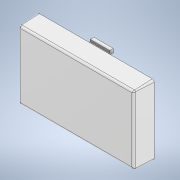
# Autodesk Inventor part: case_up
Saved by Autodesk Inventor 2022 (Build 260153000, 153)
## iProperties
Created: 2022-01-08
Part Number: case_up
Material: Пластик АБС
Document SubType Name: Modeling
Designer: Me
Density: 1.06 g/cm^3
Appearance: Гладкий — белый
Author: Me
Autodesk Inventor part; units mm, degrees
ref_plane "YZ Plane" through (0, 0, 0) normal (1, 0, 0) x (0, 1, 0)
ref_plane "XZ Plane" through (0, 0, 0) normal (0, 1, 0) x (-1, 0, 0)
ref_plane "XY Plane" through (0, 0, 0) normal (0, 0, 1) x (1, 0, 0)
sketch "Эскиз1" plane through (0, 0, 0) normal (0, 0, 1) x (1, 0, 0)
  line L0 (-29, 18) -> (29, 18)
  line L1 (30, 17) -> (30, -17)
  line L2 (29, -18) -> (-29, -18)
  line L3 (-30, -17) -> (-30, 17)
  arc A0 (-29, 18) -> (-30, 17) centre (-29, 17) ccw
  arc A1 (-30, -17) -> (-29, -18) centre (-29, -17) ccw
  arc A2 (29, -18) -> (30, -17) centre (29, -17) ccw
  arc A3 (30, 17) -> (29, 18) centre (29, 17) ccw
  point P0 (0, 0)
  point P1 (-30, 18)
  point P2 (30, 18)
  point P3 (-30, -18)
  dimension "d0" = 60
  dimension "d1" = 36
  dimension "d2" = 18
  dimension "d3" = 30
  dimension "d4" = 1
  constraints: 8 end point, 8 point on circle, 8 tangent, 6 point on line, 4 centre point, 3 equal radius, 2 parallel, 1 horizontal, 1 perpendicular
  measures "d0" distance of point (-30, 18) point (30, 18)
  measures "d1" distance of point (-30, -18) point (-30, 18)
  measures "d2" distance from line of point (0, 0) L0
  measures "d3" distance from line of point (0, 0) L1
  measures "d4" radius of A0
extrude "Выдавливание1" add sketch "Эскиз1" along normal blind 4
sketch "Эскиз3" plane through (0, 0, 4) normal (0, 0, 1) x (1, 0, 0)
  line L0 (-29, 18) -> (29, 18)
  line L1 (30, 17) -> (30, -17)
  line L2 (29, -18) -> (-29, -18)
  line L3 (-30, -17) -> (-30, 17)
  line L4 (30, -17) -> (30, 17) projected
  line L5 (-29, -18) -> (29, -18) projected
  line L6 (-30, 17) -> (-30, -17) projected
  line L7 (29, 18) -> (-29, 18) projected
  arc A0 (-29, 18) -> (-30, 17) centre (-29, 17) ccw
  arc A1 (-30, -17) -> (-29, -18) centre (-29, -17) ccw
  arc A2 (29, -18) -> (30, -17) centre (29, -17) ccw
  arc A3 (30, 17) -> (29, 18) centre (29, 17) ccw
  point P0 (0, 0)
  dimension "d7" = 0
  dimension "d8" = 0
  dimension "d9" = 0
  dimension "d10" = 0
  dimension "d11" = 1
  constraints: 8 end point, 8 point on circle, 8 tangent, 4 centre point, 3 equal radius, 2 parallel, 1 horizontal, 1 perpendicular
  measures "d7" distance between parallel lines of L4 L1
  measures "d8" distance between parallel lines of L5 L2
  measures "d9" distance between parallel lines of L6 L3
  measures "d10" distance between parallel lines of L7 L0
  measures "d11" radius of A0
extrude "Выдавливание2" add sketch "Эскиз3" along normal blind 10 draft -3
sketch "Эскиз4" plane through (0, 0, 0) normal (0, 0, -1) x (-1, 0, 0)
  line L0 (-27.5, 15.5) -> (27.5, 15.5)
  line L1 (27.5, 15.5) -> (27.5, -15.5)
  line L2 (27.5, -15.5) -> (-27.5, -15.5)
  line L3 (-27.5, -15.5) -> (-27.5, 15.5)
  point P0 (0, 0)
  dimension "d14" = 15.5
  dimension "d15" = 31
  dimension "d16" = 27.5
  dimension "d17" = 55
  constraints: 8 end point, 2 parallel, 1 horizontal, 1 perpendicular
  measures "d14" distance from line of point (0, 0) L0
  measures "d15" distance of L0.end L1.end
  measures "d16" distance from line of point (0, 0) L1
  measures "d17" distance of L0.start L0.end
extrude "Выдавливание3" cut sketch "Эскиз4" against normal blind 13 draft -3
sketch "Эскиз5" plane through (0, 0, 0) normal (0, 0, -1) x (-1, 0, 0)
  line L0 (-28.5, 16.5) -> (28.5, 16.5)
  line L1 (28.5, 16.5) -> (28.5, -16.5)
  line L2 (28.5, -16.5) -> (-28.5, -16.5)
  line L3 (-28.5, -16.5) -> (-28.5, 16.5)
  line L4 (-29, 18) -> (29, 18) projected
  line L5 (-30, -17) -> (-30, 17) projected
  line L6 (29, -18) -> (-29, -18) projected
  line L7 (30, 17) -> (30, -17) projected
  line L8 (-29, 18) -> (29, 18)
  line L9 (30, 17) -> (30, -17)
  line L10 (29, -18) -> (-29, -18)
  line L11 (-30, -17) -> (-30, 17)
  arc A0 (-29, 18) -> (-30, 17) centre (-29, 17) ccw
  arc A1 (-30, -17) -> (-29, -18) centre (-29, -17) ccw
  arc A2 (29, -18) -> (30, -17) centre (29, -17) ccw
  arc A3 (30, 17) -> (29, 18) centre (29, 17) ccw
  point P0 (0, 0)
  point P1 (29, 18)
  dimension "d20" = 1.5
  dimension "d21" = 1.5
  dimension "d22" = 1.5
  dimension "d23" = 1.5
  dimension "d24" = 0
  dimension "d25" = 0
  dimension "d26" = 0
  dimension "d27" = 0
  dimension "d28" = 1
  constraints: 16 end point, 8 point on circle, 8 tangent, 4 centre point, 4 parallel, 3 equal radius, 2 horizontal, 2 perpendicular
  measures "d20" distance between parallel lines of L4 L0
  measures "d21" distance between parallel lines of L5 L3
  measures "d22" distance between parallel lines of L6 L2
  measures "d23" distance between parallel lines of L7 L1
  measures "d24" distance between parallel lines of L4 L8
  measures "d25" distance between parallel lines of L5 L11
  measures "d26" distance between parallel lines of L6 L10
  measures "d27" distance between parallel lines of L7 L9
  measures "d28" radius of A0
extrude "Выдавливание4" cut sketch "Эскиз5" against normal blind 4
fillet "Сопряжение1" radius 1 8 edges at (-29.3365, -17.3365, 14) (-29.4759, 0, 14) (-29.3365, 17.3365, 14) (0, 17.4759, 14) (29.3365, 17.3365, 14) (29.4759, 0, 14) (29.3365, -17.3365, 14) (0, -17.4759, 14)
sketch "Эскиз6" plane through (-28.5, -16.5, 0) normal (0, -1, 0) x (1, 0, 0)
  line L0 (0, 4) -> (23.5, 4)
  line L1 (23.5, 4) -> (23.5, 0)
  line L2 (23.5, 0) -> (0, 0)
  line L3 (0, 0) -> (0, 4)
  line L4 (33.5, 4) -> (57, 4)
  line L5 (57, 4) -> (57, 0)
  line L6 (57, 0) -> (33.5, 0)
  line L7 (33.5, 0) -> (33.5, 4)
  line L8 (-0.5, 4) -> (57.5, 4) projected
  line L9 (57, 0) -> (0, 0) projected
  line L10 (0, 0) -> (0, 4) projected
  line L11 (57, 0) -> (57, 4) projected
  point P0 (28.5, 0)
  dimension "d32" = 0
  dimension "d33" = 0
  dimension "d34" = 0
  dimension "d35" = 23.5
  dimension "d36" = 0
  dimension "d37" = 23.5
  constraints: 16 end point, 4 parallel, 2 horizontal, 2 perpendicular, 2 point on line
  measures "d32" distance between parallel lines of L8 L0
  measures "d33" distance between parallel lines of L9 L2
  measures "d34" distance between parallel lines of L10 L3
  measures "d35" distance of L1.end L2.end
  measures "d36" distance between parallel lines of L11 L5
  measures "d37" distance of L5.end L6.end
extrude "Выдавливание5" cut sketch "Эскиз6" against normal through all contours L0 L1 L2 L3 | L4 L5 L6 L7
sketch "Эскиз8" plane through (-5, -16.5, 0) normal (0, -1, 0) x (1, 0, 0)
  line L0 (0, 1.9) -> (10, 1.9)
  line L1 (10, 1.9) -> (10, 0)
  line L2 (10, 0) -> (0, 0)
  line L3 (0, 0) -> (0, 1.9)
  line L4 (0, 4) -> (0, 0) projected
  line L5 (10, 0) -> (0, 0) projected
  line L6 (10, 0) -> (10, 4) projected
  point P0 (5, 0)
  dimension "d43" = 0
  dimension "d44" = 0
  dimension "d45" = 0
  dimension "d46" = 1.9
  constraints: 8 end point, 2 parallel, 1 horizontal, 1 perpendicular
  measures "d43" distance between parallel lines of L4 L3
  measures "d44" distance between parallel lines of L5 L2
  measures "d45" distance between parallel lines of L6 L1
  measures "d46" distance of L0.end L1.end
extrude "Выдавливание6" add sketch "Эскиз8" along normal blind 1
sketch "Эскиз9" plane through (-5, 16.5, 0) normal (0, 1, 0) x (1, 0, 0)
  line L0 (10, -1.9) -> (0, -1.9)
  line L1 (0, -1.9) -> (0, 0)
  line L2 (0, 0) -> (10, 0)
  line L3 (10, 0) -> (10, -1.9)
  line L4 (0, 0) -> (10, 0) projected
  line L5 (10, -4) -> (10, 0) projected
  line L6 (0, 0) -> (0, -4) projected
  point P0 (5, 0)
  dimension "d49" = 0
  dimension "d50" = 0
  dimension "d51" = 0
  dimension "d52" = 1.9
  constraints: 8 end point, 2 parallel, 1 horizontal, 1 perpendicular
  measures "d49" distance between parallel lines of L4 L2
  measures "d50" distance between parallel lines of L5 L3
  measures "d51" distance between parallel lines of L6 L1
  measures "d52" distance of L0.end L1.end
extrude "Выдавливание7" add sketch "Эскиз9" along normal blind 1
